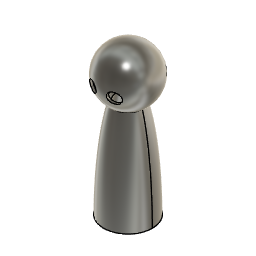
Project Overview v3 (Autodesk Fusion 360 archive; units mm, degrees)
design "Statue"
Autodesk Fusion 360 part; units mm, degrees
sketch "Sketch1" plane through (0, 0, 0) normal (0, 1, 0) x (1, 0, 0)
  line L0 (-11, 0) -> (11, 0)
  line L1 (-11, 30) -> (11, 30)
  line L2 (11, 30) -> (11, 0)
  line L3 (-11, 0) -> (-11, 30)
  ellipse E0 centre (0, 0) end of major axis (0, -55) minor radius 11
  line L4 (0, 55) -> (0, -55) construction
  line L5 (-11, 0) -> (11, 0) construction
  line L6 (0, -55) -> (0, 30)
  point P0 (0, -55)
  dimension "d22" = 55
  dimension "d23" = 30
  dimension "d24" = 22
  dimension "d25" = 22
  constraint horizontal L0
  constraint parallel L0 L1
  constraint perpendicular L0 L2
  constraint perpendicular L1 L3
  constraint coincident E0 L4.start
  constraint coincident E0 P0
  constraint coincident E0 L0.start
  constraint coincident E0 L0.end
  constraint coincident E0.centre origin
  constraint perpendicular L0 L4
  constraint coincident L0.end L2.end
  constraint coincident P0 L4.end
  constraint midpoint L1 L6.end
  measures "d22" distance of E0.centre L4.end
  measures "d23" distance of L0.end L1.end
  measures "d24" distance of L0.start L0.end
revolve "Revolve1" add sketch "Sketch1" angle 360 about axis through (0, 0, 55) along (0, 0, -1) contours L0 L1 E0 L6 | L0 E0 L6 | L1 L2 E0 picked at (3.5152, 15.2155) picked at (2.6059, -31.2309) makes body 1
sketch "Sketch2" plane through (0, 0, 0) normal (0, 1, 0) x (1, 0, 0)
  circle A0 centre (75, 0) radius 12.5
  line L0 (75, -12.5) -> (75, 12.5)
  dimension "d4" = 25
  constraint coincident A0 L0.start
  constraint coincident A0 L0.end
  constraint vertical L0
  measures "d4" diameter of A0
revolve "Revolve2" add sketch "Sketch2" angle 360 about axis through (75, 0, 12.5) along (0, 0, -1) separate body contours A0 L0 picked at (81.2506, 0.5124) makes body 2
copy_body "Body->Comp1" bodies 2 removing the originals makes body 3 in component "Component"
extrude "Extrude1" add 2 faces at (10.3, 0.8775, -30) (-4.0965, 1.9498, -30) along direction (0, 0, -1) blind 30 on bodies 1 bodies 1
combine "Combine1" operation add target body 3 tool bodies 1 body 1 seen with x (1, 0, 0) y (0, 1, 0) z (0, 0, 1) at (75, 0, -55) in component "Component"
shell "Shell1" thickness 1 removed faces 1 at (74.1841, -2.1587, -115) on bodies 3 in component "Component"
sketch "Sketch3" plane through (0, 0, 0) normal (0, 0, 1) x (1, 0, 0)
  circle A0 centre (0, 0) radius 5
  dimension "d21" = 10
  constraint coincident A0.centre origin
  measures "d21" diameter of A0
sketch "Sketch4" plane through (0, 0, 0) normal (0, 1, 0) x (1, 0, 0)
  circle A0 centre (-4.7404, -103.3418) radius 2.5
  circle A1 centre (4.9177, -103.4241) radius 2.5
  dimension "d15" = 5
  dimension "d16" = 5
  measures "d15" diameter of A0
  measures "d16" diameter of A1
extrude "Extrude2" cut sketch "Sketch4" along normal mid plane 90 contours A1 sketch seen with x (1, 0, 0) y (0, 1, 0) z (0, 0, 1) at (75, 0, -55) bodies 3 in component "Component"
extrude "Extrude3" cut sketch "Sketch4" along normal mid plane 38 contours A0 sketch seen with x (1, 0, 0) y (0, 1, 0) z (0, 0, 1) at (75, 0, -55) bodies 3 in component "Component"
extrude "Extrude4" cut 1 faces at (85.5885, 1.0433, -115) along direction (0, 0, 1) blind 10 on bodies 3 bodies 3 in component "Component"
move_body "Move1" bodies 3 to x (1, 0, 0) y (0, 1, 0) z (0, 0, 1) at (0, 0, 50) in component "Component"
sketch "Sketch5" plane through (0, 0, 0) normal (0, 1, 0) x (1, 0, 0)
  arc A0 (-2.6164, -134.9265) -> (-8, -133) centre (-8.379, -142.5447) ccw
  line L0 (0, -144) -> (0, -149.3809)
  arc A1 (8, -133) -> (2.6164, -134.9265) centre (8.379, -142.5447) ccw
  arc A2 (-2.6164, -133.9265) -> (-8, -132) centre (-8.379, -141.5447) ccw
  arc A3 (8, -132) -> (2.6164, -133.9265) centre (8.379, -141.5447) ccw
  line L1 (-8, -133) -> (-8, -132)
  line L2 (-2.6164, -134.9265) -> (-2.6164, -133.9265)
  line L3 (2.6164, -134.9265) -> (2.6164, -133.9265)
  line L4 (8, -133) -> (8, -132)
  constraint vertical L0
  constraint symmetric A0.start L0 A1.end
  constraint symmetric A0.end L0 A1.start
  constraint symmetric A0 L0 A1
  constraint vertical L1
  constraint parallel L1 L2
  constraint parallel L2 L3
  constraint parallel L3 L4
extrude "Extrude5" cut sketch "Sketch5" along normal mid plane 49 sketch seen with x (1, 0, 0) y (0, 1, 0) z (0, 0, 1) at (75, 0, -55) bodies 3 in component "Component"
sketch "Sketch6" plane through (0, 0, 0) normal (0, 1, 0) x (1, 0, 0)
  arc A0 (-2, -121.5) -> (2, -121.5) centre (0, -120) ccw
  line L0 (-2, -121.5) -> (2, -121.5)
  constraint horizontal L0
extrude "Extrude7" cut sketch "Sketch4" along normal mid plane 38 contours A1 sketch seen with x (1, 0, 0) y (0, 1, 0) z (0, 0, 1) at (75, 0, -55) bodies 3 in component "Component"
extrude "Extrude8" cut sketch "Sketch4" along normal mid plane 32 contours A0 sketch seen with x (1, 0, 0) y (0, 1, 0) z (0, 0, 1) at (75, 0, -55) bodies 3 in component "Component"
extrude "Extrude10" cut 1 faces at (85.5885, 1.0433, -55) along direction (0, 0, 1) blind 15 on bodies 3 bodies 3 in component "Component"
extrude "Extrude11" cut 1 faces at (85.5885, 1.0433, -40) along direction (0, 0, 1) blind 35 on bodies 3 bodies 3 in component "Component"
extrude "Extrude9" [rolled back] along distance 30 taper angle 0 in component "Component"
extrude "Extrude6" [suppressed] in component "Component"
component "Component" placed x (1, 0, 0) y (0, 1, 0) z (0, 0, 1) at (-75, 0, 55)

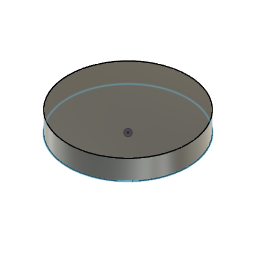
design "Button Top"
Autodesk Fusion 360 part; units mm, degrees
sketch "Sketch1" plane through (0, 0, 0) normal (0, 0, 1) x (1, 0, 0)
  circle A0 centre (0, 0) radius 15
  constraint coincident A0.centre origin
extrude "Extrude1" add sketch "Sketch1" along normal blind 5
shell "Shell1" thickness 1 removed faces 1 at (3.8315, 5.6199, 5)
sketch "Sketch2" plane through (0, 0, 1) normal (0, 0, 1) x (-1, 0, 0)
  circle A0 centre (0, 0) radius 14
  circle A1 centre (0, 0) radius 4
  circle A2 centre (0, 0) radius 3.5
  dimension "d4" = 8
  dimension "d5" = 7
  constraint concentric A0 A1
  constraint concentric A0 A2
  measures "d4" diameter of A1
  measures "d5" diameter of A2
extrude "Extrude3" add sketch "Sketch2" along normal blind 6.5 contours A1
extrude "Extrude4" add 1 faces at (-3.8184, 0.1987, 7.5) along direction (0, 0, 1) blind 2
extrude "Extrude5" cut 1 faces at (-3.8184, 0.1987, 9.5) along direction (0, 0, -1) blind 1.5
move_body "Move1" bodies 1 to x (1, 0, 0) y (0, -1, 0) z (0, 0, -1) at (0, 0, 0)
move_body "Move2" bodies 1 to x (1, 0, 0) y (0, 1, 0) z (0, 0, 1) at (0, 0, 5)
